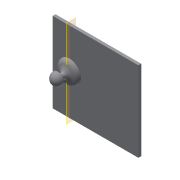
# Autodesk Inventor part: klep uitlaat
Saved by Autodesk Inventor 2019 (Build 230136000, 136)
## iProperties
Created: 2020-02-29
Part Number: klep uitlaat
Material: Generic
Document SubType Name: Modeling
Designer: stef_
Density: 1 g/cm^3
Appearance: Default
Author: stef_
Autodesk Inventor part; units mm, degrees
ref_plane "YZ Plane" through (0, 0, 0) normal (1, 0, 0) x (0, 1, 0)
ref_plane "XZ Plane" through (0, 0, 0) normal (0, 1, 0) x (-1, 0, 0)
ref_plane "XY Plane" through (0, 0, 0) normal (0, 0, 1) x (1, 0, 0)
sketch "Sketch1" plane through (0, 0, 0) normal (0, 0, 1) x (1, 0, 0)
  line L0 (74.9493, 70) -> (-74.9493, 70)
  line L1 (-74.9493, 70) -> (-74.9493, -70)
  line L2 (-74.9493, -70) -> (74.9493, -70)
  line L3 (74.9493, -70) -> (74.9493, 70)
  line L4 (86.9493, 80) -> (86.9493, -80) projected
  line L5 (-86.9493, 80) -> (86.9493, 80) projected
  line L6 (86.9493, -80) -> (-86.9493, -80) projected
  line L7 (-86.9493, -80) -> (-86.9493, 80) projected
  point P0 (0, 0)
  dimension "d0" = 12
  dimension "d1" = 12
  dimension "d2" = 10
  dimension "d3" = 10
  constraints: 8 end point, 2 parallel, 1 horizontal, 1 perpendicular
  measures "d0" distance between parallel lines of L4 L3
  measures "d1" distance between parallel lines of L7 L1
  measures "d2" distance between parallel lines of L6 L2
  measures "d3" distance between parallel lines of L5 L0
extrude "Extrusion1" add sketch "Sketch1" along normal blind 5 contours L3 L2 L1 L0
sketch "Sketch2" plane through (0, 0, 5) normal (0, 0, 1) x (1, 0, 0)
  circle A0 centre (-45.3251, 0) radius 20
  point P0 (0, 0)
  dimension "d6" = 40
  constraints: 1 centre point
  measures "d6" diameter of A0
extrude "Extrusion2" add sketch "Sketch2" along normal blind 5
ref_plane "Work Plane1" through (-45.3251, 0, 10) normal (1, 0, 0) x (0, 0, 1)
sketch "Sketch3" plane through (-45.3251, 0, 10) normal (1, 0, 0) x (0, 0, 1)
  line L0 (-5, -20) -> (0, -20) projected
  arc A0 (5.8045, -5.3429) -> (0, -20) centre (23.603, -20.8694) ccw
  arc A1 (15.5602, -10.7434) -> (5.8045, -5.3429) centre (9.0817, -10.9346) ccw
  arc A2 (15.5602, -10.7434) -> (26.3035, 0) centre (15.5602, 0) ccw
  line L1 (0, -20) -> (0, 20) projected
  line L2 (0, -20) -> (0, 0)
  line L3 (26.3035, 0) -> (0, 0)
  point P0 (-10, 0)
  constraints: 6 point on circle, 4 end point, 3 centre point, 1 midpoint, 1 perpendicular, 1 point on line
revolve "Revolution1" add sketch "Sketch3" angle 360 about axis through (-45.3251, 0, 36.3035) along (0, 0, -1)
fillet "Fillet1" radius 10 2 edges at (-31.1829, 14.1421, 10) (-59.4672, -14.1421, 10)
body "Solid1"
